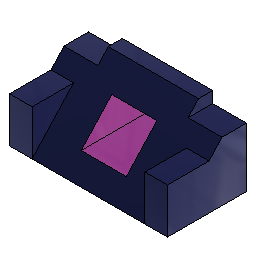
Design 17 v1 (Autodesk Fusion 360 design; units mm, degrees)
Autodesk Fusion 360 part; units mm, degrees
box "BoxPrimitive1" add length 280 width 560 height 250 placed x (0, 1, 0) y (-1, 0, 0) z (0, 0, 1) at (560, 0, 0)
sketch "Sketch2" plane through (560, 0, 0) normal (1, 0, 0) x (0, 1, 0)
  line L0 (0, 250) -> (0, 0)
  line L1 (0, 0) -> (280, 0)
  line L2 (280, 0) -> (280, 250)
  line L3 (280, 250) -> (0, 250)
  line L4 (0, 0) -> (230, 250)
  line L5 (193.2, 210) -> (280, 210)
  line L6 (147.2, 160) -> (0, 160)
  dimension "d6" = 50
  dimension "d7" = 160
  dimension "d8" = 50
  constraint coincident L0.end L1.start
  constraint coincident L3 L4.end
  constraint coincident L4 L5.start
  constraint coincident L2 L5.end
  constraint perpendicular L2 L5
  constraint coincident L4 L6.start
  constraint horizontal L6
  constraint coincident L0 L6.end
  measures "d6" distance of L2.end L4.end
  measures "d7" distance of L0.end L6
  measures "d8" vertical distance of L5.start L6.start
extrude "Extrude1" cut sketch "Sketch2" against normal blind 560 contours L0 L3 L4 L6
extrude "Extrude2" cut sketch "Sketch2" against normal blind 400 from surface at -80 contours L0 L4 L6
extrude "Extrude3" cut sketch "Sketch2" against normal blind 120 contours L2 L3 L4 L5
ref_plane "WorkPlane1" through (280, 140, 105) normal (1, 0, 0) x (0, 0, -1)
mirror "Mirror1" about plane through (280, 140, 105) normal (1, 0, 0) of "Extrude3"
sketch "Sketch3" plane through (0, 0, 0) normal (0, -0.735931, 0.677057) x (1, 0, 0)
  line L0 (120, 285.3528) -> (0, 285.3528)
  line L1 (0, 285.3528) -> (0, 217.4117)
  line L2 (0, 217.4117) -> (80, 217.4117)
  line L3 (80, 217.4117) -> (80, 0)
  line L4 (80, 0) -> (480, 0)
  line L5 (480, 0) -> (480, 217.4117)
  line L6 (480, 217.4117) -> (560, 217.4117)
  line L7 (560, 217.4117) -> (560, 285.3528)
  line L8 (560, 285.3528) -> (440, 285.3528)
  line L9 (440, 285.3528) -> (440, 339.7058)
  line L10 (440, 339.7058) -> (120, 339.7058)
  line L11 (120, 339.7058) -> (120, 285.3528)
  line L12 (360, 80) -> (200, 80)
  line L13 (200, 80) -> (200, 240)
  line L14 (200, 240) -> (360, 240)
  line L15 (360, 240) -> (360, 80)
  line L16 (360, 80) -> (200, 240) construction
  line L17 (200, 80) -> (360, 240) construction
  point P0 (280, 160)
  dimension "d18" = 160
  dimension "d19" = 160
  dimension "d20" = 80
  dimension "d21" = 120
  constraint horizontal L12
  constraint perpendicular L12 L13
  constraint parallel L12 L14
  constraint parallel L13 L15
  constraint coincident L16 P0
  constraint coincident L17 P0
  measures "d18" distance of L13.end L14.end
  measures "d19" distance of L12.end L13.end
  measures "d20" distance of L4 L12.start
  measures "d21" distance of L5 L12.start
sketch "Sketch4" plane through (0, 280, 0) normal (0, 1, 0) x (-1, 0, 0)
  line L0 (0, 210) -> (-120, 210)
  line L1 (-120, 210) -> (-120, 250)
  line L2 (-120, 250) -> (-440, 250)
  line L3 (-440, 250) -> (-440, 210)
  line L4 (-440, 210) -> (-560, 210)
  line L5 (-560, 210) -> (-560, 0)
  line L6 (-560, 0) -> (0, 0)
  line L7 (0, 0) -> (0, 210)
  line L8 (-200, 58.8745) -> (-200, 176.6234)
  line L9 (-200, 176.6234) -> (-360, 176.6234)
  line L10 (-360, 58.8745) -> (-200, 58.8745)
  line L11 (-360, 176.6234) -> (-360, 58.8745)
extrude "Extrude4" cut sketch "Sketch4" against normal blind 300 contours L8 L9 L10 L11
